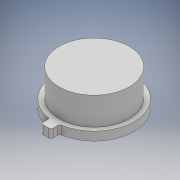
# Autodesk Inventor part: sensor
Saved by Autodesk Inventor 2018 (Build 220112000, 112)
## iProperties
Created: 2019-10-14
Part Number: sensor
Material: Generic
Document SubType Name: Modeling
Designer: jklei
Density: 1 g/cm^3
Appearance: Default
Author: jklei
Autodesk Inventor part; units mm, degrees
ref_plane "YZ Plane" through (0, 0, 0) normal (1, 0, 0) x (0, 1, 0)
ref_plane "XZ Plane" through (0, 0, 0) normal (0, 1, 0) x (-1, 0, 0)
ref_plane "XY Plane" through (0, 0, 0) normal (0, 0, 1) x (1, 0, 0)
sketch "Sketch1" plane through (0, 0, 0) normal (0, 0, 1) x (1, 0, 0)
  circle A0 centre (0, 0) radius 4.6
  dimension "d0" = 9.2
  constraints: 1 centre point, 1 coincident
  measures "d0" diameter of A0
extrude "Extrusion1" add sketch "Sketch1" along normal blind 1
sketch "Sketch2" plane through (0, 0, 1) normal (0, 0, 1) x (1, 0, 0)
  circle A0 centre (0, 0) radius 4.05
  dimension "d3" = 8.1
  constraints: 1 centre point, 1 coincident
  measures "d3" diameter of A0
extrude "Extrusion2" add sketch "Sketch2" along normal blind 3.2
sketch "Sketch3" plane through (0, 0, 0) normal (0, 0, -1) x (-1, 0, 0)
  line L0 (0, 0) -> (0, -4.6024)
  line L1 (0, -4.6024) -> (-0.5737, -4.5641)
  circle A0 centre (0, 0) radius 4.6 projected
  line L2 (-0.5737, -4.5641) -> (0.5763, -4.5638)
  line L3 (0.5763, -4.5638) -> (0.5766, -5.5638)
  line L4 (0.5766, -5.5638) -> (-0.5734, -5.5641)
  line L5 (-0.5734, -5.5641) -> (-0.5737, -4.5641)
  dimension "d6" = 0.575
  dimension "d7" = 1.15
  dimension "d8" = 1
  constraints: 12 end point, 3 perpendicular, 2 point on circle, 1 vertical
  measures "d6" distance of L0.end L1.end
  measures "d7" distance of L1.end L2.end
  measures "d8" distance of L2.end L3.end
extrude "Extrusion3" add sketch "Sketch3" against normal blind 1 contours A0 L3 L4 L5 L1
fillet "Fillet1" radius 0.25 4 edges at (0.5737, -4.5641, 0.5) (0.5734, -5.5641, 0.5) (-0.5763, -4.5638, 0.5) (-0.5766, -5.5638, 0.5)
body "Solid1"
